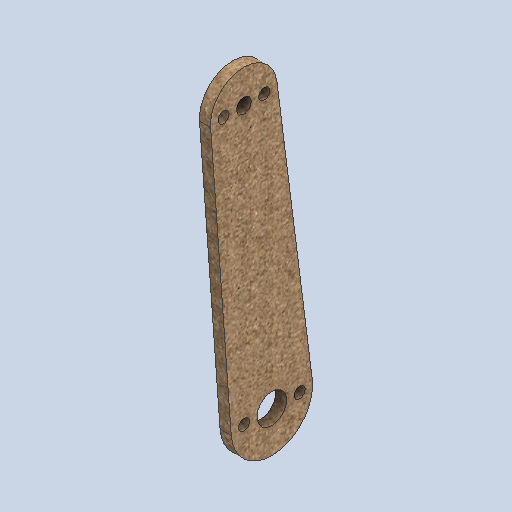
# Autodesk Inventor part: roller-hand-v2-MDF-link-1
Saved by Autodesk Inventor 2025.1 (Build 291241000, 241)
## iProperties
Created: 2024-10-06
Part Number: roller-hand-v2-MDF-link-1
Material: MDF 中密度繊維ボード
Document SubType Name: Modeling
Designer: haruy
Density: 0.8 g/cm^3
Appearance: ダンボール - 段ボール紙
Author: haruy
Autodesk Inventor part; units mm, degrees
ref_plane "YZ Plane" through (0, 0, 0) normal (1, 0, 0) x (0, 1, 0)
ref_plane "XZ Plane" through (0, 0, 0) normal (0, 1, 0) x (-1, 0, 0)
ref_plane "XY Plane" through (0, 0, 0) normal (0, 0, 1) x (1, 0, 0)
derived "roller-hand-v2-Sketch-Base.ipt"
sketch "スケッチ1" plane through (200, 0, 0) normal (1, 0, 0) x (0, 1, 0)
  circle A0 centre (0, 0) radius 4
  circle A1 centre (15.5291, -57.9555) radius 9
  circle A2 centre (7.2469, -27.0459) radius 16
  circle A3 centre (27.4423, -44.1692) radius 2
  circle A4 centre (74.6196, 7.5445) radius 2
  line L0 (74.6196, 7.5445) -> (0, 0) construction
  line L1 (74.6196, 7.5445) -> (27.4423, -44.1692)
  line L2 (0, 0) -> (27.4423, -44.1692) construction
  line L3 (0, 0) -> (15.5291, -57.9555) construction
  circle A5 centre (0, -184.4555) radius 117.5
  line L4 (155.3866, 15.5445) -> (-185.0808, 15.5445)
  circle A6 centre (0, 0) radius 60 construction
  line L5 (0, 0) -> (28.2083, -52.9555) construction
  circle A7 centre (0, 0) radius 52 construction
  circle A8 centre (36.6749, -36.864) radius 4 construction
  line L6 (74.6196, 7.5445) -> (36.6749, -36.864) construction
  circle A9 centre (27.4423, -44.1692) radius 9
  circle A10 centre (74.6196, 7.5445) radius 9
  circle A11 centre (15.5291, -57.9555) radius 12.5
  circle A12 centre (0, 0) radius 11
  circle A13 centre (7.2469, -27.0459) radius 9
  circle A14 centre (15.5291, -57.9555) radius 16
  circle A15 centre (7.2469, -27.0459) radius 16
  line L7 (20.4525, -18.0119) -> (34.8704, -39.0876)
  circle A16 centre (15.5291, -57.9555) radius 12.5
  line L8 (26.3809, -64.1595) -> (35.2556, -48.636)
  line L9 (-7.6622, -32.8526) -> (3.8814, -62.492)
  circle A17 centre (0, 0) radius 11
  line L10 (73.9533, 16.5198) -> (-0.8143, 10.9698)
  line L11 (1.398, -10.9108) -> (75.7634, -1.3826)
  line L12 (9.946, 4.6986) -> (21.7139, -20.2116) construction
  line L13 (-10.9628, -0.9039) -> (-8.699, -28.3607)
  circle A18 centre (74.6196, 7.5445) radius 5.5
  circle A19 centre (74.6196, 13.0445) radius 1.5
  line L14 (74.6196, 7.5445) -> (74.6196, 13.0445)
  circle A20 centre (74.6196, 2.0445) radius 1.5
  circle A21 centre (0, 0) radius 7.5
  circle A22 centre (0, 7.5) radius 1.5
  circle A23 centre (0, -7.5) radius 1.5
  line L15 (0, -184.4555) -> (117.5, -184.4555)
  dimension "d1" = 11
  dimension "d7" = 15
  dimension "d2" = 3
  dimension "d5" = 360
  dimension "d8" = 3
  dimension "d11" = 360
  measures "d2" diameter of A19
  measures "d8" diameter of A22
sketch "スケッチ2" plane through (0, 200, 0) normal (0, 1, 0) x (-1, 0, 0)
  line L0 (0, 0) -> (280, 0)
  line L1 (280, 0) -> (280, -18)
  line L2 (280, -18) -> (0, -18)
  line L3 (0, -18) -> (0, 0)
  line L4 (-5, 116.1253) -> (-8, 116.1253)
  line L5 (-8, 116.1253) -> (-8, -29.5691)
  line L6 (-8, -29.5691) -> (-5, -29.5691)
  line L7 (-5, -29.5691) -> (-5, 116.1253)
  line L8 (-5, 52.6222) -> (66.2, 52.6222)
  line L9 (66.2, 52.6222) -> (66.2, 20.6222)
  line L10 (66.2, 20.6222) -> (-5, 20.6222)
  line L11 (-5, 20.6222) -> (-5, 52.6222)
  line L12 (-5, 46.6222) -> (-9, 46.6222)
  line L13 (-9, 46.6222) -> (-9, 26.6222)
  line L14 (-9, 26.6222) -> (-5, 26.6222)
  line L15 (-5, 26.6222) -> (-5, 46.6222)
  line L16 (-9, 39.6222) -> (-23.8, 39.6222)
  line L17 (-23.8, 39.6222) -> (-23.8, 33.6222)
  line L18 (-23.8, 33.6222) -> (-9, 33.6222)
  line L19 (-9, 33.6222) -> (-9, 39.6222)
  line L20 (-14, 45.0445) -> (-20, 45.0445)
  line L21 (-20, 45.0445) -> (-20, 23.8894)
  line L22 (-20, 23.8894) -> (-14, 23.8894)
  line L23 (-14, 23.8894) -> (-14, 45.0445)
  line L24 (-20, 50.3109) -> (-26, 50.3109)
  line L25 (-26, 50.3109) -> (-26, 18.3109)
  line L26 (-26, 18.3109) -> (-20, 18.3109)
  line L27 (-20, 18.3109) -> (-20, 50.3109)
  line L28 (15, 0) -> (15, -18)
  line L29 (15, -4.3972) -> (-26, -4.3972)
  line L30 (-26, -4.3972) -> (-26, -16.3972)
  line L31 (-26, -16.3972) -> (15, -16.3972)
  line L32 (15, -16.3972) -> (15, -4.3972)
  line L33 (-14.8, 155.9564) -> (-17.8, 155.9564)
  line L34 (-17.8, 155.9564) -> (-17.8, 85.4399)
  line L35 (-17.8, 85.4399) -> (-14.8, 85.4399)
  line L36 (-14.8, 85.4399) -> (-14.8, 155.9564)
  line L37 (-21.6284, 147.0378) -> (100.6034, 147.0378)
  line L38 (100.6034, 147.0378) -> (100.6034, 143.0378)
  line L39 (100.6034, 143.0378) -> (-21.6284, 143.0378)
  line L40 (-21.6284, 143.0378) -> (-21.6284, 147.0378)
ref_plane "作業平面1" through (200, 0, 0) normal (1, 0, 0) x (0, 1, 0)
ref_plane "作業平面2" through (0, 200, 0) normal (0, 1, 0) x (-1, 0, 0)
extrude "押し出し1" add sketch "スケッチ1" along normal blind 3 contours A12 | L11 A12 L10 L4 A10 L1 | L1 A10 L11 | A10 L4 | L10 A10 L4 | A10 L4 | A4 L14 A19 A18 A20 L1 | A4 L1 A18 A19 L14 | A21 A23 A22
